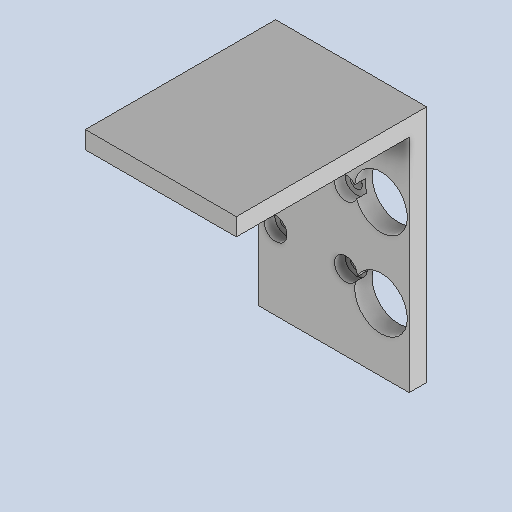
# Autodesk Inventor part: TS_Adapter_Greifer_int
Saved by Autodesk Inventor 2025.1 (Build 291241000, 241)
## iProperties
Created: 2025-06-16
Part Number: TS_Adapter_Greifer_int
Material: Generisch
Document SubType Name: Modeling
Designer: tino
Density: 1 g/cm^3
Appearance: Vorgabe
Author: tino
Autodesk Inventor part; units mm, degrees
ref_plane "YZ Plane" through (0, 0, 0) normal (1, 0, 0) x (0, 1, 0)
ref_plane "XZ Plane" through (0, 0, 0) normal (0, 1, 0) x (-1, 0, 0)
ref_plane "XY Plane" through (0, 0, 0) normal (0, 0, 1) x (1, 0, 0)
sketch "Skizze1" plane through (0, 0, 0) normal (0, 0, 1) x (1, 0, 0)
  line L0 (-21.5, 27.1) -> (21.5, 27.1)
  line L1 (21.5, 27.1) -> (21.5, -27.1)
  line L2 (21.5, -27.1) -> (-21.5, -27.1)
  line L3 (-21.5, -27.1) -> (-21.5, 27.1)
  line L4 (0, 37.94) -> (0, -37.94) projected
  line L5 (-30.1, 0) -> (30.1, 0) projected
  point P0 (0, 0)
  dimension "d0" = 43
  dimension "d1" = 54.2
  dimension "d46" = 21.5
  dimension "d47" = 27.1
  constraints: 8 end point, 2 parallel, 1 horizontal, 1 perpendicular
  measures "d0" distance of L1.end L2.end
  measures "d1" distance of L2.end L0.start
  measures "d46" distance between parallel lines of L3 L4
  measures "d47" distance between parallel lines of L5 L2
extrude "Extrusion1" add sketch "Skizze1" along normal blind 63
sketch "Skizze2" plane through (0, 0, 63) normal (0, 0, 1) x (1, 0, 0)
  line L0 (-21.5, -27.1) -> (21.5, -27.1) projected
  line L1 (-16.5, -27.1) -> (26.5, -27.1)
  line L2 (26.5, -27.1) -> (26.5, 22.1)
  line L3 (26.5, 22.1) -> (-16.5, 22.1)
  line L4 (-16.5, 22.1) -> (-16.5, -27.1)
  line L5 (-21.5, 27.1) -> (-21.5, -27.1) projected
  line L6 (21.5, 27.1) -> (-21.5, 27.1) projected
  point P0 (0, 0)
  point P1 (24, -27.1)
  dimension "d4" = 43
  dimension "d6" = 5
  dimension "d69" = 5
  constraints: 8 end point, 2 parallel, 1 horizontal, 1 perpendicular, 1 point on line
  measures "d4" distance of L2.end L3.end
  measures "d6" distance between parallel lines of L6 L3
  measures "d69" distance between parallel lines of L5 L4
extrude "Extrusion2" cut sketch "Skizze2" against normal through all
sketch "Skizze4" plane through (-21.5, 22.1, 0) normal (0, 1, 0) x (1, 0, 0)
  line L0 (43, -63) -> (0, -63) projected
  line L1 (43, 0) -> (0, 0) projected
  line L2 (0, -63) -> (43, -63) construction
  line L3 (43, 0) -> (43, -63) construction
  line L4 (5, 0) -> (5, -63) projected
  point P0 (21.5, 0)
  point P1 (25, -41.5)
  point P2 (5, -41.5)
  point P3 (25, -21.5)
  point P4 (5, -21.5)
  point P5 (43, -63)
  dimension "d9" = 20
  dimension "d17" = 63
  dimension "d64" = 21.5
  dimension "d71" = 20
  dimension "d72" = 43
  constraints: 2 horizontal alignment, 2 vertical alignment, 1 point on line
  measures "d9" distance of point (25, -21.5) point (25, -41.5)
  measures "d17" distance of L1.end L0.end
  measures "d64" distance from line of L1 point (5, -21.5)
  measures "d71" distance of point (25, -41.5) point (5, -41.5)
  measures "d72" distance of L1.start L1.end
hole "Bohrung1" at (3.5, 22.1, 41.5) at (-16.5, 22.1, 41.5) at (3.5, 22.1, 21.5) at (-16.5, 22.1, 21.5) direction (0, 1, 0) diameter 3.4 end through all counterbore diameter 6.5 counterbore depth 3
sketch "Skizze6" plane through (-21.5, 27.1, 0) normal (0, 1, 0) x (1, 0, 0)
  line L0 (43, -63) -> (0, -63) projected
  line L1 (43, 0) -> (0, 0) projected
  line L2 (21.5, 12.6) -> (21.5, -75.6) projected
  circle A0 centre (5, -41.5) radius 1.7 projected
  point P0 (21.5, 0)
  point P1 (15, -44)
  point P2 (15, -19)
  dimension "d48" = 25
  dimension "d49" = 63
  dimension "d50" = 19
  dimension "d76" = 10
  constraints: 1 vertical alignment
  measures "d48" distance of point (15, -19) point (15, -44)
  measures "d49" distance between parallel lines of L0 L1
  measures "d50" distance from line of L1 point (15, -19)
  measures "d76" horizontal distance of A0.centre point (15, -44)
hole "Bohrung4" at (-6.5, 27.1, 44) at (-6.5, 27.1, 19) direction (0, -1, 0) diameter 5 depth 2.5
sketch "Skizze9" plane through (0, 0, 63) normal (0, 0, 1) x (1, 0, 0)
  line L0 (21.5, 27.1) -> (-21.5, 27.1) projected
  line L1 (-21.5, -27.1) -> (21.5, -27.1)
  line L2 (21.5, -27.1) -> (21.5, 27.1)
  line L3 (21.5, 27.1) -> (-21.5, 27.1)
  line L4 (-21.5, 27.1) -> (-21.5, -27.1)
  line L5 (-21.5, 27.1) -> (-21.5, -27.1) projected
  line L6 (-21.5, -27.1) -> (-16.5, -27.1) projected
  point P0 (0, 0)
  constraints: 8 end point, 2 collinear, 2 parallel, 1 horizontal, 1 perpendicular
extrude "Extrusion5" add sketch "Skizze9" along normal blind 5
sketch "Skizze11" plane through (-21.5, -27.1, 0) normal (-1, 0, 0) x (0, 0, 1)
  line L0 (0, 54.2) -> (0, 0) projected
  line L1 (63, 0) -> (68, 0) projected
  line L2 (48, 49.2) -> (63, 0)
  line L3 (0, 54.2) -> (68, 54.2) projected
  line L4 (0, 0) -> (68, 0) projected
  line L5 (68, 54.2) -> (68, 0) projected
  line L6 (48, 49.2) -> (0, 49.2)
  point P0 (0, 27.1)
  dimension "d84" = 5
  dimension "d87" = 20
  constraints: 4 end point, 1 horizontal, 1 point on line
  measures "d84" distance from line of L3 L2.start
  measures "d87" distance from line of L2.start L5
extrude "Extrusion7" cut sketch "Skizze11" against normal blind 5 contours L6 L2 L4 L0
sketch "Skizze12" plane through (-21.5, 27.1, 0) normal (0, 1, 0) x (1, 0, 0)
  line L0 (43, -68) -> (0, -68) projected
  line L1 (43, 0) -> (43, -68) projected
  point P0 (21.5, 0)
  point P1 (35, -43)
  point P2 (35, -18)
  dimension "d88" = 25
  dimension "d89" = 8
  dimension "d90" = 25
  measures "d88" distance from line of point (35, -43) L0
  measures "d89" distance from line of L1 point (35, -43)
  measures "d90" distance of point (35, -43) point (35, -18)
hole "Bohrung5" at (13.5, 27.1, 43) at (13.5, 27.1, 18) direction (0, -1, 0) diameter 15 end through all
equation "\"d46\" = 0.5 * d0"
equation "\"d47\" = 0.5 * d1"
equation "\"d6\" = d5"
equation "\"d50\" = -0.5 * d48 + 0.5 * d49"
equation "\"d5\" = 5"
